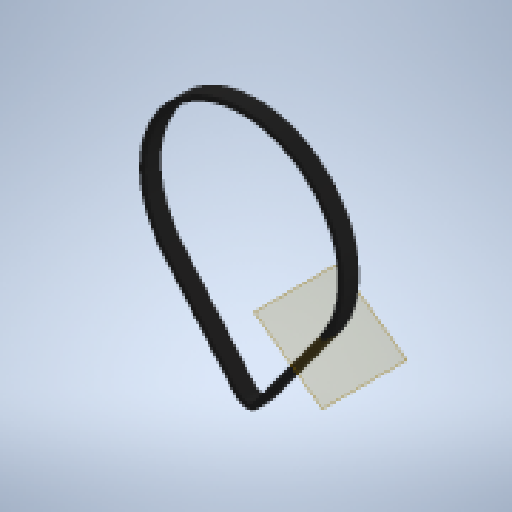
# Autodesk Inventor part: belt
Saved by Autodesk Inventor 2024 (Build 280153000, 153)
## iProperties
Created: 2024-02-15
Part Number: belt
Material: Generic
Document SubType Name: Modeling
Designer: fabiancastano
Density: 1 g/cm^3
Appearance: Default
Author: fabiancastano
Autodesk Inventor part; units mm, degrees
ref_plane "YZ Plane" through (0, 0, 0) normal (1, 0, 0) x (0, 1, 0)
ref_plane "XZ Plane" through (0, 0, 0) normal (0, 1, 0) x (-1, 0, 0)
ref_plane "XY Plane" through (0, 0, 0) normal (0, 0, 1) x (1, 0, 0)
sketch "Sketch1" plane through (0, 0, 0) normal (0, 0, 1) x (1, 0, 0)
  arc A0 (21.0123, -15.4044) -> (-20.0568, -16.8099) centre (-0.0744, 0.0265) ccw
  arc A1 (-1.3604, -38.9999) -> (3.8767, -38.8206) centre (1.1877, -36.8529) ccw
  line L0 (-1.3604, -38.9999) -> (-20.0568, -16.8099)
  line L1 (3.8767, -38.8206) -> (21.0123, -15.4044)
  point P0 (0, 0)
  constraints: 4 end point, 4 point on circle, 4 tangent, 2 centre point
ref_plane "Work Plane1" through (21.0123, -15.4044, 0) normal (0.5906, 0.807, 0) x (-0.807, 0.5906, 0)
sketch "Sketch2" plane through (21.0123, -15.4044, 0) normal (0.5906, 0.807, 0) x (-0.807, 0.5906, 0)
  line L0 (1.0661, 2.0494) -> (-0.4231, 2.0494)
  line L1 (-0.4231, 2.0494) -> (-0.4231, -2.0661)
  line L2 (-0.4231, -2.0661) -> (1.0661, -2.0661)
  line L3 (1.0661, -2.0661) -> (1.0661, 2.0494)
  point P0 (26.054, 0)
  constraints: 8 end point, 2 parallel, 1 horizontal, 1 perpendicular
sweep "Sweep1" add profiles "Sketch2" path "Sketch1"
body "Solid1"
